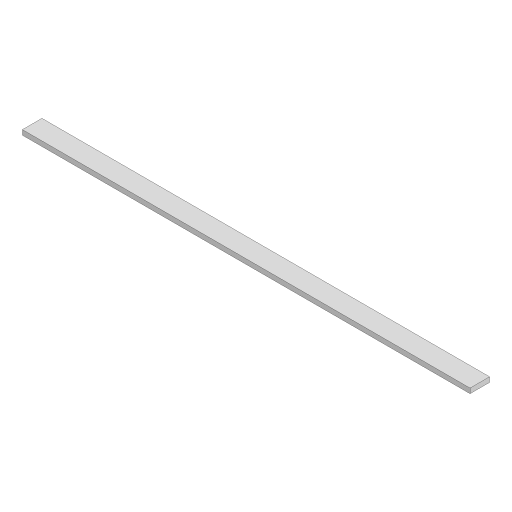
# Autodesk Inventor part: boxsectiontest
Saved by Autodesk Inventor 2024 (Build 280153000, 153)
## iProperties
Created: 2024-02-23
Part Number: boxsectiontest
Material: Generic
Document SubType Name: Modeling
Designer: Frank
Density: 1 g/cm^3
Appearance: Default
Author: Frank
Autodesk Inventor part; units mm, degrees
ref_plane "YZ Plane" through (0, 0, 0) normal (1, 0, 0) x (0, 1, 0)
ref_plane "XZ Plane" through (0, 0, 0) normal (0, 1, 0) x (-1, 0, 0)
ref_plane "XY Plane" through (0, 0, 0) normal (0, 0, 1) x (1, 0, 0)
sketch "Sketch1" plane through (0, 0, 0) normal (1, 0, 0) x (0, 1, 0)
  line L0 (0, 0) -> (65, 0)
  line L1 (65, 0) -> (65, -262)
  line L2 (65, -262) -> (0, -262)
  line L3 (0, -262) -> (0, 0)
  dimension "d0" = 65
  dimension "d1" = 262
  constraints: 8 end point, 2 parallel, 1 horizontal, 1 perpendicular
  measures "d0" distance of L1.end L2.end
  measures "d1" distance of L0.end L1.end
extrude "Extrusion1" add sketch "Sketch1" along normal blind 6000
body "Solid1"
